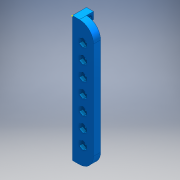
# Autodesk Inventor part: bottomSideFrame
Saved by Autodesk Inventor 2016 (Build 200138000, 138)
## iProperties
Created: 2016-06-05
Part Number: bottomSideFrame
Material: ABS Plastic
Document SubType Name: Modeling
Designer: hesaon
Density: 1.06 g/cm^3
Appearance: Smooth - White
Author: hesaon
Autodesk Inventor part; units mm, degrees
ref_plane "YZ Plane" through (0, 0, 0) normal (1, 0, 0) x (0, 1, 0)
ref_plane "XZ Plane" through (0, 0, 0) normal (0, 1, 0) x (-1, 0, 0)
ref_plane "XY Plane" through (0, 0, 0) normal (0, 0, 1) x (1, 0, 0)
sketch "Sketch1" plane through (0, 0, 0) normal (0, 1, 0) x (-1, 0, 0)
  line L0 (0, 0) -> (-30, 0)
  line L1 (-30, -20) -> (-30, -158)
  line L2 (-10, -178) -> (0, -178)
  line L3 (0, -178) -> (0, 0)
  arc A0 (-10, 0) -> (-30, -20) centre (-10, -20) ccw
  line L4 (-10, -20) -> (-30, -20) construction
  line L5 (-10, -20) -> (-10, 0) construction
  arc A1 (-30, -158) -> (-10, -178) centre (-10, -158) ccw
  line L6 (-10, -158) -> (-10, -178) construction
  line L7 (-10, -158) -> (-30, -158) construction
  dimension "d2" = 90
  dimension "d3" = 20
  dimension "d4" = 10
  dimension "d6" = 90
  dimension "d10" = 20
  dimension "d11" = 20
  dimension "d12" = 178
  constraints: 16 end point, 4 point on circle, 3 parallel, 2 centre point, 1 horizontal, 1 perpendicular, 1 point on line
  measures "d2" angle of L5 L4
  measures "d3" distance of L5.end L4.start
  measures "d4" horizontal distance of L4.start L0.start
  measures "d6" angle of L7 L6
  measures "d10" horizontal distance of L5.end L1.start
  measures "d11" horizontal distance of L1.end L2.start
  measures "d12" distance of L2.end L0.start
extrude "Extrusion1" add sketch "Sketch1" along normal blind 10
sketch "Sketch2" plane through (0, 0, 0) normal (0, -1, 0) x (1, 0, 0)
  line L0 (-10, -89) -> (40, -89)
  line L1 (15, -188) -> (15, 10)
  circle A0 centre (15, -89) radius 3.1
  circle A1 centre (15, -68) radius 3.1
  circle A2 centre (15, -47) radius 3.1
  circle A3 centre (15, -26) radius 3.1
  circle A4 centre (15, -110) radius 3.1
  circle A5 centre (15, -131) radius 3.1
  circle A6 centre (15, -152) radius 3.1
  point P0 (0, 0)
  dimension "d16" = 198
  dimension "d17" = 15
  dimension "d18" = 6.2
  dimension "d19" = 6.2
  dimension "d20" = 6.2
  dimension "d21" = 6.2
  dimension "d22" = 6.2
  dimension "d23" = 6.2
  dimension "d24" = 6.2
  dimension "d25" = 21
  dimension "d26" = 21
  dimension "d27" = 21
  dimension "d28" = 21
  dimension "d29" = 21
  dimension "d30" = 21
  dimension "d31" = 89
  dimension "d32" = 10
  dimension "d33" = 50
  dimension "d34" = 10
  constraints: 7 centre point, 2 end point, 1 horizontal, 1 midpoint, 10 other
  measures "d16" distance of point (15, 10) point (15, -188)
  measures "d17" horizontal distance of point (0, 0) point (15, 10)
  measures "d18" diameter of A0
  measures "d19" diameter of A1
  measures "d20" diameter of A2
  measures "d21" diameter of A3
  measures "d22" diameter of A4
  measures "d23" diameter of A5
  measures "d24" diameter of A6
  measures "d25" distance of A4.centre A0.centre
  measures "d26" distance of A5.centre A4.centre
  measures "d27" distance of A5.centre A6.centre
  measures "d28" distance of A1.centre A0.centre
  measures "d29" distance of A1.centre A2.centre
  measures "d30" distance of A3.centre A2.centre
  measures "d31" vertical distance of point (0, 0) L0.start
  measures "d32" vertical distance of point (0, 0) point (15, 10)
  measures "d33" distance of L0.end L0.start
  measures "d34" horizontal distance of L0.start point (0, 0)
extrude "Extrusion2" cut sketch "Sketch2" against normal up to next
sketch "Sketch3" plane through (0, 10, 0) normal (0, 1, 0) x (1, 0, 0)
  line L0 (0, 178) -> (0, 0) projected
  line L1 (0, 0) -> (10, 0)
  line L2 (10, 0) -> (10, 10)
  line L3 (10, 10) -> (0, 10)
  line L4 (0, 10) -> (0, 0)
  line L5 (0, 178) -> (0, 0) projected
  line L6 (0, 0) -> (10, 0) projected
  line L7 (0, 52) -> (10, 52)
  line L8 (10, 52) -> (10, 62)
  line L9 (10, 62) -> (0, 62)
  line L10 (0, 62) -> (0, 52)
  line L11 (10, 118) -> (0, 118)
  line L12 (0, 118) -> (0, 128)
  line L13 (0, 128) -> (10, 128)
  line L14 (10, 128) -> (10, 118)
  dimension "d39" = 10
  dimension "d40" = 10
  dimension "d41" = 10
  dimension "d42" = 10
  dimension "d43" = 42
  dimension "d44" = 10
  dimension "d45" = 10
  dimension "d46" = 56
  constraints: 24 end point, 6 parallel, 4 collinear, 3 horizontal, 3 perpendicular
  measures "d39" distance of L3.end L2.end
  measures "d40" distance of L2.end L1.end
  measures "d41" distance of L9.end L8.end
  measures "d42" distance of L8.end L7.end
  measures "d43" distance between parallel lines of L7 L3
  measures "d44" distance of L12.end L13.end
  measures "d45" distance of L11.end L12.end
  measures "d46" distance between parallel lines of L9 L11
extrude "Extrusion3" add sketch "Sketch3" along normal blind 10
sketch "Sketch4" plane through (0, 10, 0) normal (0, 1, 0) x (1, 0, 0)
  line L0 (10, 62) -> (0, 62)
  line L1 (0, 62) -> (0, 118)
  line L2 (0, 118) -> (10, 118)
  line L3 (10, 118) -> (10, 62)
  line L4 (10, 62) -> (0, 62) projected
  line L5 (0, 118) -> (10, 118) projected
  line L6 (0, 118) -> (0, 62) projected
  point P0 (0, 0)
  dimension "d49" = 10
  constraints: 8 end point, 3 collinear, 2 parallel, 1 horizontal, 1 perpendicular
  measures "d49" distance of L1.end L2.end
extrude "Extrusion4" add sketch "Sketch4" along normal blind 10
sketch "Sketch5" plane through (0, 10, 0) normal (0, 1, 0) x (1, 0, 0)
  line L0 (10, 74) -> (25, 74)
  line L1 (25, 74) -> (25, 83)
  line L2 (25, 83) -> (10, 83)
  line L3 (10, 83) -> (10, 74)
  circle A0 centre (15, 89) radius 3.1 projected
  circle A1 centre (15, 89) radius 3.1 projected
  circle A2 centre (15, 89) radius 3.1 projected
  circle A3 centre (15, 68) radius 3.1 projected
  circle A4 centre (15, 68) radius 3.1 projected
  circle A5 centre (15, 110) radius 3.1 projected
  line L4 (10, 128) -> (10, 52) projected
  line L5 (10, 95) -> (25, 95)
  line L6 (25, 95) -> (25, 104)
  line L7 (25, 104) -> (10, 104)
  line L8 (10, 104) -> (10, 95)
  point P0 (0, 0)
  dimension "d52" = 15
  dimension "d53" = 9
  dimension "d54" = 6
  dimension "d55" = 15
  dimension "d56" = 9
  dimension "d57" = 6
  constraints: 16 end point, 4 parallel, 2 collinear, 2 horizontal, 2 perpendicular
  measures "d52" distance of L2.end L1.end
  measures "d53" distance of L1.end L0.end
  measures "d54" distance from line of L2 A0.centre
  measures "d55" distance of L7.end L6.end
  measures "d56" distance of L6.end L5.end
  measures "d57" distance from line of L5 A0.centre
extrude "Extrusion5" add sketch "Sketch5" along normal blind 10 contours L3 L2 L1 L0 | L7 L6 L5 L4
chamfer "Chamfer1" distance 10 angle 45 2 edges at (25, 20, -78.5) (25, 20, -99.5)
hole "Hole1" at (10, 15, -5) direction (-1, 0, 0) diameter 4.3 end up to face face through (0, 3.3333, -76.6667) facing (-1, 0, 0)
hole "Hole2" at (10, 15, -57) direction (-1, 0, 0) diameter 4.3 end up to face face through (0, 3.3333, -76.6667) facing (-1, 0, 0)
hole "Hole3" at (10, 15, -123) direction (-1, 0, 0) diameter 4.3 end up to face face through (0, 3.3333, -76.6667) facing (-1, 0, 0)
sketch "Sketch6" plane through (0, 10, 0) normal (0, 1, 0) x (1, 0, 0)
  line L0 (0, 168) -> (10, 168)
  line L1 (10, 168) -> (10, 178)
  line L2 (10, 178) -> (0, 178)
  line L3 (0, 178) -> (0, 168)
  line L4 (10, 178) -> (0, 178) projected
  line L5 (0, 178) -> (0, 128) projected
  point P0 (0, 0)
  dimension "d90" = 10
  dimension "d91" = 10
  constraints: 8 end point, 2 collinear, 2 parallel, 1 horizontal, 1 perpendicular
  measures "d90" distance of L2.end L1.end
  measures "d91" distance of L1.end L0.end
extrude "Extrusion6" add sketch "Sketch6" along normal blind 10
hole "Hole4" at (10, 15, -173) direction (-1, 0, 0) diameter 4.3 end up to face face through (0, 3.3333, -76.6667) facing (-1, 0, 0)
sketch "Sketch7" plane through (0, 0, 0) normal (0, -1, 0) x (1, 0, 0)
  point P0 (0, 0)
sketch "Sketch8" plane through (0, 0, 0) normal (0, -1, 0) x (1, 0, 0)
  circle A0 centre (15, -26) radius 3.1 projected
  line L0 (15, -19.9956) -> (20.2, -22.9978)
  line L1 (20.2, -22.9978) -> (20.2, -29.0022)
  line L2 (20.2, -29.0022) -> (15, -32.0044)
  line L3 (15, -32.0044) -> (9.8, -29.0022)
  line L4 (9.8, -29.0022) -> (9.8, -22.9978)
  line L5 (9.8, -22.9978) -> (15, -19.9956)
  circle A1 centre (15, -47) radius 3.1 projected
  line L6 (20.2, -43.9978) -> (20.2, -50.0022)
  line L7 (20.2, -50.0022) -> (15, -53.0044)
  line L8 (15, -53.0044) -> (9.8, -50.0022)
  line L9 (9.8, -50.0022) -> (9.8, -43.9978)
  line L10 (9.8, -43.9978) -> (15, -40.9956)
  line L11 (15, -40.9956) -> (20.2, -43.9978)
  circle A2 centre (15, -68) radius 3.1 projected
  line L12 (20.2, -64.9978) -> (20.2, -71.0022)
  line L13 (20.2, -71.0022) -> (15, -74.0044)
  line L14 (15, -74.0044) -> (9.8, -71.0022)
  line L15 (9.8, -71.0022) -> (9.8, -64.9978)
  line L16 (9.8, -64.9978) -> (15, -61.9956)
  line L17 (15, -61.9956) -> (20.2, -64.9978)
  circle A3 centre (15, -89) radius 3.1 projected
  line L18 (15, -82.9956) -> (20.2, -85.9978)
  line L19 (20.2, -85.9978) -> (20.2, -92.0022)
  line L20 (20.2, -92.0022) -> (15, -95.0044)
  line L21 (15, -95.0044) -> (9.8, -92.0022)
  line L22 (9.8, -92.0022) -> (9.8, -85.9978)
  line L23 (9.8, -85.9978) -> (15, -82.9956)
  circle A4 centre (15, -110) radius 3.1 projected
  circle A5 centre (15, -131) radius 3.1 projected
  line L24 (20.2, -127.9978) -> (20.2, -134.0022)
  line L25 (20.2, -134.0022) -> (15, -137.0044)
  line L26 (15, -137.0044) -> (9.8, -134.0022)
  line L27 (9.8, -134.0022) -> (9.8, -127.9978)
  line L28 (9.8, -127.9978) -> (15, -124.9956)
  line L29 (15, -124.9956) -> (20.2, -127.9978)
  circle A6 centre (15, -152) radius 3.1 projected
  line L30 (20.2, -148.9978) -> (20.2, -155.0022)
  line L31 (20.2, -155.0022) -> (15, -158.0044)
  line L32 (15, -158.0044) -> (9.8, -155.0022)
  line L33 (9.8, -155.0022) -> (9.8, -148.9978)
  line L34 (9.8, -148.9978) -> (15, -145.9956)
  line L35 (15, -145.9956) -> (20.2, -148.9978)
  line L36 (20.2, -106.9978) -> (20.2, -113.0022)
  line L37 (20.2, -113.0022) -> (15, -116.0044)
  line L38 (15, -116.0044) -> (9.8, -113.0022)
  line L39 (9.8, -113.0022) -> (9.8, -106.9978)
  line L40 (9.8, -106.9978) -> (15, -103.9956)
  line L41 (15, -103.9956) -> (20.2, -106.9978)
  point P0 (0, 0)
  point P1 (9.8, -26)
  point P2 (9.8, -47)
  point P3 (9.8, -68)
  point P4 (9.8, -89)
  point P5 (9.8, -152)
  point P6 (9.8, -110)
  point P7 (9.8, -131)
  dimension "d103" = 10.4
  dimension "d104" = 10.4
  dimension "d105" = 10.4
  dimension "d106" = 10.4
  dimension "d107" = 10.4
  dimension "d108" = 10.4
  dimension "d109" = 10.4
  constraints: 84 end point, 8 coincident, 7 midpoint, 7 vertical alignment, 91 other
  measures "d103" distance between parallel lines of L1 L4
  measures "d104" distance between parallel lines of L30 L33
  measures "d105" distance between parallel lines of L37 L40
  measures "d106" distance between parallel lines of L25 L28
  measures "d107" distance between parallel lines of L20 L23
  measures "d108" distance between parallel lines of L13 L16
  measures "d109" distance between parallel lines of L7 L10
extrude "Extrusion7" cut sketch "Sketch8" against normal blind 5
body "Solid1"
